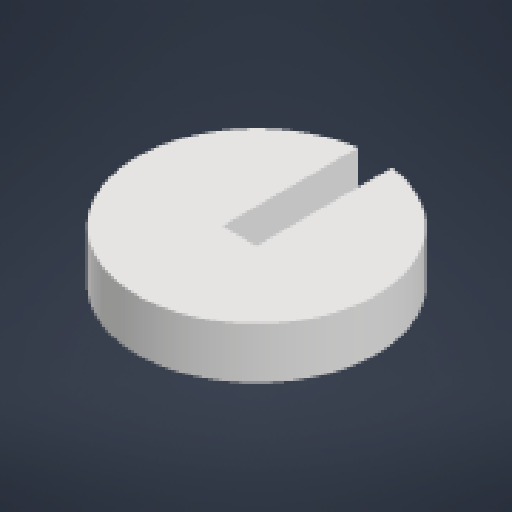
# Autodesk Inventor part: 1kg Disc Mass
Saved by Autodesk Inventor 2023.1 (Build 271208000, 208)
## iProperties
Created: 2022-12-07
Part Number: 1kg Disc Mass
Material: Generic
Document SubType Name: Modeling
Designer: aubrey-work
Density: 1 g/cm^3
Appearance: Default
Author: aubrey-work
Autodesk Inventor part; units mm, degrees
ref_plane "YZ Plane" through (0, 0, 0) normal (1, 0, 0) x (0, 1, 0)
ref_plane "XZ Plane" through (0, 0, 0) normal (0, 1, 0) x (-1, 0, 0)
ref_plane "XY Plane" through (0, 0, 0) normal (0, 0, 1) x (1, 0, 0)
sketch "Sketch1" plane through (0, 0, 0) normal (0, 1, 0) x (-1, 0, 0)
  circle A0 centre (0, 0) radius 44.45
  dimension "d0" = 88.9
  constraints: 1 centre point, 1 coincident
  measures "d0" diameter of A0
extrude "Extrusion1" add sketch "Sketch1" along normal blind 19.05
sketch "Sketch2" plane through (0, 19.05, 0) normal (0, 1, 0) x (1, 0, 0)
  line L0 (6.35, -6.35) -> (-6.35, -6.35)
  line L1 (-6.35, -6.35) -> (-6.35, 57.15)
  line L2 (-6.35, 57.15) -> (6.35, 57.15)
  line L3 (6.35, 57.15) -> (6.35, -6.35)
  line L4 (6.35, -6.35) -> (-6.35, 57.15) construction
  line L5 (-6.35, -6.35) -> (6.35, 57.15) construction
  point P0 (0, 0)
  point P1 (0, 25.4)
  point P2 (0, -6.35)
  dimension "d3" = 12.7
  dimension "d4" = 63.5
  dimension "d5" = 6.35
  dimension "d6" = 0
  constraints: 12 end point, 3 midpoint, 2 parallel, 1 horizontal, 1 perpendicular
  measures "d3" distance of L1.end L2.end
  measures "d4" distance of L0.end L1.end
  measures "d5" distance of point (0, 0) point (0, -6.35)
  measures "d6" horizontal distance of point (0, 25.4) point (0, 0)
extrude "Extrusion2" cut sketch "Sketch2" against normal blind 19.05
body "Solid1"
